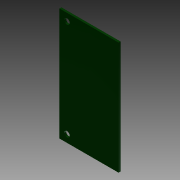
# Autodesk Inventor part: AddonPCB01
Saved by Autodesk Inventor 2013 (Build 170138000, 138)
## iProperties
Created: 2014-04-13
Part Number: AddonPCB01
Material: PCB(1)
Document SubType Name: Modeling
Designer: spichelh
Density: 1 g/cm^3
Author: spichelh
Autodesk Inventor part; units mm, degrees
ref_plane "YZ Plane" through (0, 0, 0) normal (1, 0, 0) x (0, 1, 0)
ref_plane "XZ Plane" through (0, 0, 0) normal (0, 1, 0) x (-1, 0, 0)
ref_plane "XY Plane" through (0, 0, 0) normal (0, 0, 1) x (1, 0, 0)
sketch "Sketch1" plane through (0, 0, 0) normal (0, 0, 1) x (1, 0, 0)
  line L0 (-15, -28.575) -> (15, -28.575)
  line L1 (15, -28.575) -> (15, 28.575)
  line L2 (15, 28.575) -> (-15, 28.575)
  line L3 (-15, 28.575) -> (-15, -28.575)
  line L4 (-15, -28.575) -> (15, 28.575) construction
  line L5 (15, -28.575) -> (-15, 28.575) construction
  circle A0 centre (-11.19, 24.765) radius 1.4
  line L6 (-15, 0) -> (15, 0) construction
  line L7 (0, 28.575) -> (0, -28.575) construction
  circle A1 centre (-11.19, -24.765) radius 1.4
  point P0 (0, 0)
  dimension "d2" = 30
  dimension "d4" = 57.15
  dimension "d6" = 2.8
  dimension "d21" = 3.81
  dimension "d22" = 3.81
  dimension "d23" = 3.81
  dimension "d24" = 3.81
  constraints: 16 end point, 6 midpoint, 2 centre point, 2 parallel, 1 horizontal, 1 perpendicular, 1 symmetric about line, 1 other
  measures "d2" distance of L1.end L2.end
  measures "d4" distance of L0.end L1.end
  measures "d6" diameter of A1
  measures "d21" distance from line of L2 A0.centre
  measures "d22" distance from line of L3 A0.centre
  measures "d23" distance from line of L3 A1.centre
  measures "d24" distance from line of L0 A1.centre
extrude "Extrusion1" add sketch "Sketch1" along normal blind 1
body "Solid1"
